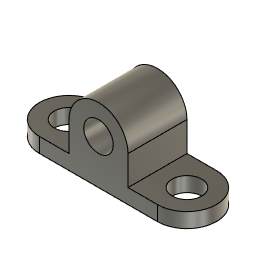
A4 shape (Autodesk Fusion 360 design; units mm, degrees)
Autodesk Fusion 360 part; units mm, degrees
note: some values were not read from the file. Set by a fixed rule: which sketch regions a step uses.
sketch "Sketch1" plane through (0, 0, 0) normal (0, 0, 1) x (1, 0, 0)
  line L0 (40, 20) -> (-40, 20)
  line L1 (-40, 20) -> (-40, -20)
  line L2 (-40, -20) -> (40, -20)
  line L3 (40, -20) -> (40, 20)
  line L4 (40, 20) -> (-40, -20) construction
  line L5 (-40, 20) -> (40, -20) construction
  line L6 (-20, 20) -> (-20, -20) construction
  line L7 (20, 20) -> (20, -20) construction
  circle A0 centre (40, 0) radius 20
  circle A1 centre (40, 0) radius 10
  circle A2 centre (-40, 0) radius 10
  circle A3 centre (-40, 0) radius 20
  dimension "d1" = 80
  dimension "d2" = 40
  dimension "d3" = 40
  dimension "d4" = 20
  dimension "d5" = 40
  dimension "d6" = 20
  dimension "d7" = 20
  dimension "d8" = 40
  constraint horizontal L0
  constraint perpendicular L0 L1
  constraint parallel L0 L2
  constraint parallel L1 L3
  constraint coincident L4 origin
  constraint coincident L5 origin
  constraint coincident L0 L6.start
  constraint coincident L2 L6.end
  constraint perpendicular L2 L6
  constraint coincident L2 L7.end
  constraint perpendicular L2 L7
  constraint midpoint L3 A0.centre
  constraint concentric A0 A1
  constraint midpoint L1 A2.centre
  constraint concentric A2 A3
  measures "d1" distance of L1.end L2.end
  measures "d2" distance of L0.end L1.end
  measures "d3" distance of L6 L7
  measures "d4" distance of L3 L7
  measures "d5" diameter of A0
  measures "d6" diameter of A1
  measures "d7" diameter of A2
  measures "d8" diameter of A3
extrude "Extrude1" add sketch "Sketch1" along normal blind 10 contours L0 L2 A0 A3 | L3 A0 A1 | L3 A0 A1 | L1 A2 A3 | L1 A2 A3
sketch "Sketch2" plane through (0, 0, 0) normal (0, 1, 0) x (1, 0, 0)
  line L0 (-40, -10) -> (-20, -10) construction
  line L1 (-20, -10) -> (20, -10)
  line L2 (20, -10) -> (20, -30)
  line L3 (20, -30) -> (-20, -30)
  line L4 (-20, -30) -> (-20, -10)
  circle A0 centre (0, -30) radius 10
  circle A1 centre (0, -30) radius 20
  dimension "d11" = 20
  dimension "d12" = 40
  dimension "d13" = 20
  dimension "d14" = 20
  dimension "d15" = 40
  constraint horizontal L0
  constraint horizontal L1
  constraint vertical L2
  constraint horizontal L3
  constraint vertical L4
  constraint midpoint L3 A0.centre
  constraint concentric A0 A1
  measures "d11" distance of L0.start L0.end
  measures "d12" distance of L0.end L1.end
  measures "d13" distance of L0.end L3.end
  measures "d14" diameter of A0
  measures "d15" diameter of A1
extrude "Extrude2" add sketch "Sketch2" along normal mid plane 40 contours L1 L4 A1 | L1 L2 A1 | L3 A0 A1 | L3 A0 A1
